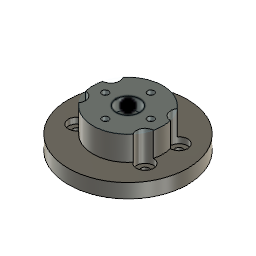
5f6ab101-cd6e-40bf-9284-99c555d6d14d (Autodesk Fusion 360 design; units mm, degrees)
part number: 2026-05-18-16-40-51-722
Autodesk Fusion 360 part; units mm, degrees
note: some values were not read from the file. Set by a fixed rule: which sketch regions a step uses.
sketch "スケッチ1" plane through (0, 0, 0) normal (0, 0, 1) x (1, 0, 0)
  circle A0 centre (0, 0) radius 21
  dimension "d1" = 42
  constraint coincident A0.centre origin
  measures "d1" diameter of A0
extrude "押し出し1" add sketch "スケッチ1" along normal blind 5
sketch "スケッチ2" plane through (0, 0, 5) normal (0, 0, 1) x (-1, 0, 0)
  circle A0 centre (0, 0) radius 21
  circle A1 centre (0, 0) radius 12.3
  dimension "d4" = 24.6
  constraint coincident A0.centre A1.centre
  measures "d4" diameter of A1
extrude "押し出し2" add sketch "スケッチ2" along normal blind 8.6 contours A1
sketch "スケッチ3" plane through (0, 0, 13.6) normal (0, 0, 1) x (-1, 0, 0)
  circle A0 centre (0, 0) radius 12.3
  circle A1 centre (0, 0) radius 4.15
  dimension "d7" = 8.3
  constraint coincident A0.centre A1.centre
  measures "d7" diameter of A1
extrude "押し出し3" cut sketch "スケッチ3" against normal blind 4.2 contours A1
sketch "スケッチ4" plane through (0, 0, 0) normal (0, 0, -1) x (1, 0, 0)
  circle A0 centre (0, 0) radius 21
  circle A1 centre (0, 0) radius 8
  circle A2 centre (0, -8) radius 1.15
  circle A3 centre (8, 0) radius 1.15
  circle A4 centre (0, 8) radius 1.15
  circle A5 centre (-8, 0) radius 1.15
  dimension "d10" = 16
  dimension "d11" = 2.3
  dimension "d12" = 2.3
  dimension "d13" = 2.3
  dimension "d14" = 2.3
  constraint coincident A0.centre A1.centre
  constraint coincident A1 A2.centre
  constraint coincident A1 A3.centre
  constraint coincident A1 A4.centre
  constraint coincident A1 A5.centre
  measures "d10" diameter of A1
  measures "d11" diameter of A2
  measures "d12" diameter of A3
  measures "d13" diameter of A4
  measures "d14" diameter of A5
extrude "押し出し4" cut sketch "スケッチ4" against normal through all contours A1 A3 | A1 A3 | A1 A4 | A1 A4 | A1 A2 | A1 A2 | A1 A5 | A1 A5
sketch "スケッチ5" plane through (0, 0, 0) normal (0, 0, -1) x (1, 0, 0)
  circle A0 centre (8, 0) radius 1.15
  circle A1 centre (0, 8) radius 1.15
  circle A2 centre (0, -8) radius 1.15
  circle A3 centre (-8, 0) radius 1.15
  circle A4 centre (0, 0) radius 21
  line L0 (12, -6) -> (-12, -6)
  line L1 (-12, -6) -> (-12, 6)
  line L2 (-12, 6) -> (12, 6)
  line L3 (12, 6) -> (12, -6)
  circle A5 centre (12, -6) radius 1.4
  circle A6 centre (-12, -6) radius 1.4
  circle A7 centre (12, 6) radius 1.4
  circle A8 centre (-12, 6) radius 1.4
  dimension "d16" = 24
  dimension "d17" = 12
  dimension "d18" = 12
  dimension "d19" = 6
  dimension "d20" = 2.8
  dimension "d21" = 2.8
  dimension "d22" = 2.8
  dimension "d23" = 2.8
  constraint horizontal L0
  constraint vertical L1
  constraint horizontal L2
  constraint vertical L3
  constraint coincident L0.start L3.end
  constraint coincident L0.end L1.start
  constraint coincident L2.end L3.start
  constraint coincident L1.end L2.start
  measures "d16" distance of L0.start L0.end
  measures "d17" distance of L0.start L2.end
  measures "d18" distance of A4.centre L3
  measures "d19" distance of A4.centre L0
  measures "d20" diameter of A5
  measures "d21" diameter of A6
  measures "d22" diameter of A7
  measures "d23" diameter of A8
extrude "押し出し5" cut sketch "スケッチ5" against normal through all contours L0 L1 A6 | L0 L1 A6 | L0 L3 A5 | L0 L3 A5 | L1 L2 A8 | L1 L2 A8 | L2 L3 A7 | L2 L3 A7
sketch "スケッチ6" plane through (0, 0, 0) normal (0, 0, -1) x (1, 0, 0)
  circle A0 centre (0, 0) radius 21
  circle A1 centre (-8, 0) radius 1.15
  circle A2 centre (0, -8) radius 1.15
  circle A3 centre (0, 8) radius 1.15
  circle A4 centre (8, 0) radius 1.15
  circle A5 centre (-12, 6) radius 1.4
  circle A6 centre (12, -6) radius 1.4
  circle A7 centre (-12, -6) radius 1.4
  circle A8 centre (12, 6) radius 1.4
  circle A9 centre (-8, 0) radius 2.25
  circle A10 centre (0, 8) radius 2.25
  circle A11 centre (8, 0) radius 2.25
  circle A12 centre (0, -8) radius 2.25
  dimension "d25" = 4.5
  dimension "d26" = 4.5
  dimension "d27" = 4.5
  dimension "d28" = 4.5
  constraint concentric A1 A9
  constraint concentric A3 A10
  constraint concentric A4 A11
  constraint concentric A2 A12
  measures "d25" diameter of A9
  measures "d26" diameter of A10
  measures "d27" diameter of A11
  measures "d28" diameter of A12
extrude "押し出し6" cut sketch "スケッチ6" against normal blind 12.1 contours A9 | A10 | A11 | A12
sketch "スケッチ7" plane through (0, 0, 13.6) normal (0, 0, 1) x (-1, 0, 0)
  circle A0 centre (12, -6) radius 3
  circle A1 centre (12, 6) radius 3
  circle A2 centre (-12, -6) radius 3
  circle A3 centre (-12, 6) radius 3
  dimension "d31" = 6
  dimension "d32" = 6
  dimension "d33" = 6
  dimension "d34" = 6
  measures "d31" diameter of A0
  measures "d32" diameter of A1
  measures "d33" diameter of A2
  measures "d34" diameter of A3
extrude "押し出し7" cut sketch "スケッチ7" against normal blind 10.7
equation "d18 = d16 / 2"
equation "d19 = d17 / 2"
